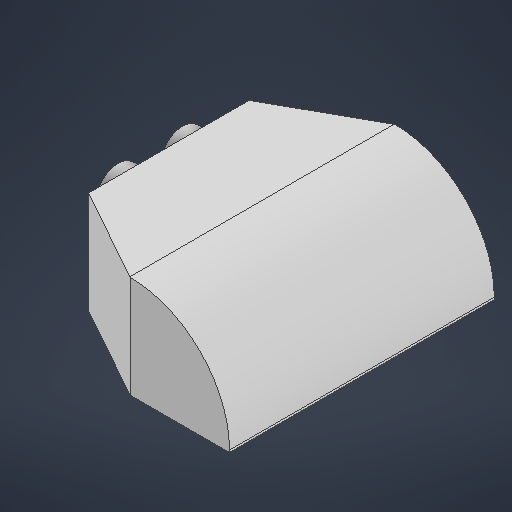
# Autodesk Inventor part: Airbox
Saved by Autodesk Inventor 2027 (Build 310192000, 192)
## iProperties
Created: 2026-09-12
Part Number: Airbox
Material: Generic
Document SubType Name: Modeling
Designer: W Ahmad
Density: 1 g/cm^3
Appearance: Default
Author: W Ahmad
Autodesk Inventor part; units mm, degrees
ref_plane "YZ Plane" through (0, 0, 0) normal (1, 0, 0) x (0, 1, 0)
ref_plane "XZ Plane" through (0, 0, 0) normal (0, 1, 0) x (-1, 0, 0)
ref_plane "XY Plane" through (0, 0, 0) normal (0, 0, 1) x (1, 0, 0)
sketch "Sketch1" plane through (0, 0, 0) normal (0, 1, 0) x (-1, 0, 0)
  line L0 (57.15, 152.4) -> (-57.15, 152.4)
  line L1 (-57.15, 152.4) -> (-57.15, -152.4)
  line L2 (-57.15, -152.4) -> (57.15, -152.4)
  line L3 (57.15, -152.4) -> (57.15, 152.4)
  line L4 (57.15, 152.4) -> (165.1, 152.4)
  line L5 (165.1, 152.4) -> (165.1, -152.4)
  line L6 (165.1, -152.4) -> (57.15, -152.4)
  line L7 (57.15, -152.4) -> (57.15, 152.4)
  line L8 (57.15, -152.4) -> (57.15, -92.4)
  line L9 (57.15, -92.4) -> (165.1, -92.4)
  line L10 (57.15, -152.4) -> (165.1, -92.4)
  line L11 (57.15, 152.4) -> (57.15, 92.4)
  line L12 (57.15, 92.4) -> (165.1, 92.4)
  line L13 (57.15, 152.4) -> (165.1, 92.4)
  point P0 (0, 0)
  point P1 (57.15, 0)
  point P2 (0, -152.4)
  dimension "d0" = 304.8
  dimension "d1" = 114.3
  dimension "d2" = 107.95
  dimension "d3" = 60
  dimension "d4" = 60
  constraints: 28 end point, 5 parallel, 4 perpendicular, 4 point on line, 2 horizontal, 2 midpoint, 1 horizontal alignment, 1 vertical alignment
  measures "d0" distance of L2.end L0.start
  measures "d1" distance of L1.end L2.end
  measures "d2" distance of L0.start L4.end
  measures "d3" distance of L6.end L8.end
  measures "d4" distance of L0.start L11.end
extrude "Extrusion1" add sketch "Sketch1" along normal blind 117.5 contours L3 L2 L1 L0 | L13 L12 L3 | L12 L5 L9 L3 | L9 L10 L3
fillet "Fillet1" radius 115 1 edges at (57.15, 117.5, 0)
sketch "Sketch2" plane through (-165.1, 0, -92.4) normal (-1, 0, 0) x (0, 0, 1)
  line L0 (55.275, 83.975) -> (55.275, 72.025) construction
  line L1 (30.65, 83.975) -> (30.65, 72.025)
  line L2 (79.9, 72.025) -> (79.9, 83.975)
  arc A0 (79.9, 83.975) -> (30.65, 83.975) centre (55.275, 83.975) ccw
  arc A1 (30.65, 72.025) -> (79.9, 72.025) centre (55.275, 72.025) ccw
  line L3 (129.525, 83.975) -> (129.525, 72.025) construction
  line L4 (104.9, 83.975) -> (104.9, 72.025)
  line L5 (154.15, 72.025) -> (154.15, 83.975)
  arc A2 (154.15, 83.975) -> (104.9, 83.975) centre (129.525, 83.975) ccw
  arc A3 (104.9, 72.025) -> (154.15, 72.025) centre (129.525, 72.025) ccw
  line L6 (92.4, 0) -> (92.4, 114.666) construction
  line L7 (0, 117.5) -> (184.8, 117.5) projected
  line L8 (107.3, 83.975) -> (107.3, 72.025)
  arc A4 (107.3, 72.025) -> (151.75, 72.025) centre (129.525, 72.025) ccw
  line L9 (151.75, 72.025) -> (151.75, 83.975)
  arc A5 (151.75, 83.975) -> (107.3, 83.975) centre (129.525, 83.975) ccw
  line L10 (33.05, 83.975) -> (33.05, 72.025)
  arc A6 (33.05, 72.025) -> (77.5, 72.025) centre (55.275, 72.025) ccw
  line L11 (77.5, 72.025) -> (77.5, 83.975)
  arc A7 (77.5, 83.975) -> (33.05, 83.975) centre (55.275, 83.975) ccw
  point P0 (55.275, 78)
  point P1 (129.525, 78)
  point P2 (129.525, 47.4)
  point P3 (129.525, 108.6)
  point P4 (129.525, 106.2)
  point P5 (55.275, 47.4)
  point P6 (55.275, 108.6)
  dimension "d8" = 12.5
  dimension "d9" = 61.2
  dimension "d10" = 49.25
  dimension "d12" = 2.4
  dimension "d14" = 8.9
  dimension "d15" = 12.5
  dimension "d16" = 61.2
  dimension "d17" = 49.25
  dimension "d18" = 8.9
  dimension "d19" = 2.4
  constraints: 26 end point, 21 point on circle, 8 centre point, 8 tangent, 5 parallel, 2 midpoint, 2 vertical, 6 other
  measures "d8" distance between parallel lines of L6 L4
  measures "d9" distance of point (129.525, 47.4) point (129.525, 108.6)
  measures "d10" distance between parallel lines of L5 L4
  measures "d12" radial gap between concentric circles of A2 A5
  measures "d14" distance from line of L7 point (129.525, 108.6)
  measures "d15" distance between parallel lines of L2 L6
  measures "d16" distance of point (55.275, 47.4) point (55.275, 108.6)
  measures "d17" distance between parallel lines of L2 L1
  measures "d18" distance from line of point (55.275, 108.6) L7
  measures "d19" radial gap between concentric circles of A0 A7
extrude "Extrusion2" add sketch "Sketch2" along normal blind 21.5
body "Solid1"
